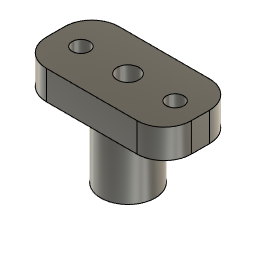
Temp Probe Holder v1 (Autodesk Fusion 360 design; units mm, degrees)
Autodesk Fusion 360 part; units mm, degrees
sketch "Sketch Baseline" plane through (0, 0, 0) normal (0, 0, 1) x (1, 0, 0)
  line L0 (0, 0) -> (40, 0)
  line L1 (40, 0) -> (40, -20)
  line L2 (40, -20) -> (0, -20)
  line L3 (0, -20) -> (0, 0)
  circle A0 centre (20, -10) radius 3
  line L4 (0, -10) -> (40, -10) construction
  line L5 (20, 0) -> (20, -20) construction
  line L6 (27.5, -17.5) -> (12.5, -17.5)
  line L7 (12.5, -17.5) -> (12.5, -2.5)
  line L8 (12.5, -2.5) -> (27.5, -2.5)
  line L9 (27.5, -2.5) -> (27.5, -17.5)
  line L10 (27.5, -17.5) -> (12.5, -2.5) construction
  line L11 (12.5, -17.5) -> (27.5, -2.5) construction
  circle A1 centre (20, -10) radius 2
  point P0 (20, -10)
  point P1 (20, -10)
  point P2 (20, -20)
  point P3 (33, -10)
  point P4 (7, -10)
  dimension "d1" = 40
  dimension "d2" = 20
  dimension "d3" = 6
  dimension "d6" = 15
  dimension "d7" = 15
  dimension "d38" = 7
  constraint horizontal L0
  constraint vertical L1
  constraint horizontal L2
  constraint vertical L3
  constraint coincident L0.start L3.end
  constraint midpoint L3 L4.start
  constraint midpoint L1 L4.end
  constraint midpoint L0 L5.start
  constraint midpoint L2 P2
  constraint midpoint P1 L4
  constraint horizontal L6
  constraint perpendicular L6 L7
  constraint parallel L6 L8
  constraint parallel L7 L9
  constraint coincident L10 P1
  constraint coincident L11 P1
  constraint coincident P1 P0
  constraint coincident P2 L5.end
  constraint coincident L4 P3
  constraint symmetric L5 P3 P4
  measures "d1" distance of L0.start L0.end
  measures "d2" distance of L0.start L2.end
  measures "d3" diameter of A0
  measures "d6" distance of L7.end L8.end
  measures "d7" distance of L6.end L7.end
  measures "d38" distance of L1 P3
extrude "Extrude1" add sketch "Sketch Baseline" against normal blind 4 contours L0 L1 L2 L3 | L6 L7 L8 L9
extrude "Extrude4" add sketch "Sketch Baseline" against normal blind 22 contours L6 L7 L8 L9
extrude "Extrude5" add sketch "Sketch Baseline" along normal blind 2 from surface at -22 contours A0
extrude "Extrude6" [suppressed]
extrude "Extrude7" add sketch "Sketch Baseline" against normal blind 2 from surface at -18 contours A0
chamfer "Chamfer1" distance 1 angle 45 1 edges at (18.1353, -9.2768, -18) measured on face at (22.6481, -10.2484, -18)
fillet "Fillet1" radius 7.5 8 edges at (40, -20, -2) (0, -20, -2) (0, 0, -2) (40, 0, -2) (27.5, -2.5, -13) (12.5, -2.5, -13) (12.5, -17.5, -13) (27.5, -17.5, -13)
sketch "Sketch Screw Holes" plane through (0, 0, -4) normal (0, 0, -1) x (1, 0, 0)
  circle A0 centre (20, 10) radius 7.5
  arc A1 (32.5, 0) -> (40, 7.5) centre (32.5, 7.5) ccw
  line L0 (40, 7.5) -> (40, 12.5)
  arc A2 (40, 12.5) -> (32.5, 20) centre (32.5, 12.5) ccw
  line L1 (32.5, 20) -> (7.5, 20)
  arc A3 (7.5, 20) -> (0, 12.5) centre (7.5, 12.5) ccw
  line L2 (0, 12.5) -> (0, 7.5)
  arc A4 (0, 7.5) -> (7.5, 0) centre (7.5, 7.5) ccw
  line L3 (7.5, 0) -> (32.5, 0)
  point P0 (7, 10)
  point P1 (33, 10)
extrude "Extrude8" add 1 faces at (31.8227, -5.6838, 0) along direction (0, 0, 1) blind 4
hole "Hole2" at (7, -10, -4) at (33, -10, -4) direction (0, 0, 1) diameter 4.8 depth 14 tip angle 180 counterbore diameter 9.6 counterbore depth 4
equation "d1 = BaseLength"
equation "d2 = BaseWidth"
equation "d3 = TubeDiameter"
equation "d6 = SupportDim"
equation "d7 = SupportDim"
equation "d9 = -TubeWallThickness"
equation "d32 = SupportDim / 2"
equation "SupportDim = 15 mm"
equation "BaseLength = 40 mm"
equation "BaseWidth = BaseLength / 2"
equation "TubeDiameter = 6 mm"
equation "TubeWallThickness = 1 mm"
named bodies: "Temp Probe Holder"
